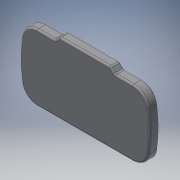
# Autodesk Inventor part: back cover
Saved by Autodesk Inventor 2019 (Build 230136000, 136)
## iProperties
Created: 2021-03-14
Part Number: back cover
Material: Generic
Document SubType Name: Modeling
Designer: Vijay
Density: 1 g/cm^3
Appearance: Default
Author: Vijay
Autodesk Inventor part; units mm, degrees
ref_plane "YZ Plane" through (0, 0, 0) normal (1, 0, 0) x (0, 1, 0)
ref_plane "XZ Plane" through (0, 0, 0) normal (0, 1, 0) x (-1, 0, 0)
ref_plane "XY Plane" through (0, 0, 0) normal (0, 0, 1) x (1, 0, 0)
sketch "Sketch1" plane through (0, 0, 0) normal (0, 0, 1) x (1, 0, 0)
  line L0 (-31.6571, 36.2117) -> (-28.1216, 39.7473) projected
  line L1 (-28.1216, 39.7473) -> (28.1216, 39.7473) projected
  line L2 (28.1216, 39.7473) -> (31.6571, 36.2117) projected
  arc A0 (31.6571, 36.2117) -> (35.1926, 34.7473) centre (35.1926, 39.7473) ccw projected
  line L3 (35.1926, 34.7473) -> (54.241, 34.7473) projected
  arc A1 (70.0672, 21.0991) -> (54.241, 34.7473) centre (54.241, 18.7473) ccw projected
  arc A2 (70.0672, -23.1161) -> (70.0672, 21.0991) centre (-78.6991, -1.0085) ccw projected
  arc A3 (54.241, -36.7642) -> (70.0672, -23.1161) centre (54.241, -20.7642) ccw projected
  line L4 (54.241, -36.7642) -> (-54.241, -36.7642) projected
  arc A4 (-70.0672, -23.1161) -> (-54.241, -36.7642) centre (-54.241, -20.7642) ccw projected
  arc A5 (-70.0672, 21.0991) -> (-70.0672, -23.1161) centre (78.6991, -1.0085) ccw projected
  arc A6 (-54.241, 34.7473) -> (-70.0672, 21.0991) centre (-54.241, 18.7473) ccw projected
  line L5 (-54.241, 34.7473) -> (-35.1926, 34.7473) projected
  arc A7 (-35.1926, 34.7473) -> (-31.6571, 36.2117) centre (-35.1926, 39.7473) ccw projected
  arc A8 (-27.7074, 41.7473) -> (-29.8287, 40.8686) centre (-27.7074, 38.7473) ccw projected
  line L6 (-29.8287, 40.8686) -> (-33.0713, 37.6259) projected
  arc A9 (-35.1926, 36.7473) -> (-33.0713, 37.6259) centre (-35.1926, 39.7473) ccw projected
  line L7 (-35.1926, 36.7473) -> (-54.241, 36.7473) projected
  arc A10 (-54.241, 36.7473) -> (-72.0455, 21.3931) centre (-54.241, 18.7473) ccw projected
  arc A11 (-72.0455, 21.3931) -> (-72.0455, -23.41) centre (78.6991, -1.0085) ccw projected
  arc A12 (-72.0455, -23.41) -> (-54.241, -38.7642) centre (-54.241, -20.7642) ccw projected
  line L8 (-54.241, -38.7642) -> (54.241, -38.7642) projected
  arc A13 (54.241, -38.7642) -> (72.0455, -23.41) centre (54.241, -20.7642) ccw projected
  arc A14 (72.0455, -23.41) -> (72.0455, 21.3931) centre (-78.6991, -1.0085) ccw projected
  arc A15 (72.0455, 21.3931) -> (54.241, 36.7473) centre (54.241, 18.7473) ccw projected
  line L9 (54.241, 36.7473) -> (35.1926, 36.7473) projected
  arc A16 (33.0713, 37.6259) -> (35.1926, 36.7473) centre (35.1926, 39.7473) ccw projected
  line L10 (33.0713, 37.6259) -> (29.8287, 40.8686) projected
  arc A17 (29.8287, 40.8686) -> (27.7074, 41.7473) centre (27.7074, 38.7473) ccw projected
  line L11 (27.7074, 41.7473) -> (-27.7074, 41.7473) projected
  line L12 (54.241, 32.7473) -> (35.1926, 32.7473) projected
  arc A18 (68.0889, 20.8051) -> (54.241, 32.7473) centre (54.241, 18.7473) ccw projected
  arc A19 (68.0889, -22.8221) -> (68.0889, 20.8051) centre (-78.6991, -1.0085) ccw projected
  arc A20 (54.241, -34.7642) -> (68.0889, -22.8221) centre (54.241, -20.7642) ccw projected
  line L13 (-54.241, -34.7642) -> (54.241, -34.7642) projected
  arc A21 (-68.0889, -22.8221) -> (-54.241, -34.7642) centre (-54.241, -20.7642) ccw projected
  arc A22 (-68.0889, 20.8051) -> (-68.0889, -22.8221) centre (78.6991, -1.0085) ccw projected
  arc A23 (-54.241, 32.7473) -> (-68.0889, 20.8051) centre (-54.241, 18.7473) ccw projected
  line L14 (-35.1926, 32.7473) -> (-54.241, 32.7473) projected
  arc A24 (-35.1926, 32.7473) -> (-30.2429, 34.7975) centre (-35.1926, 39.7473) ccw projected
  line L15 (-27.2931, 37.7473) -> (-30.2429, 34.7975) projected
  line L16 (27.2931, 37.7473) -> (-27.2931, 37.7473) projected
  line L17 (30.2429, 34.7975) -> (27.2931, 37.7473) projected
  arc A25 (30.2429, 34.7975) -> (35.1926, 32.7473) centre (35.1926, 39.7473) ccw projected
  line L18 (-28.1216, 39.7473) -> (28.1216, 39.7473) projected
  line L19 (-31.6571, 36.2117) -> (-28.1216, 39.7473) projected
  arc A26 (-35.1926, 34.7473) -> (-31.6571, 36.2117) centre (-35.1926, 39.7473) ccw projected
  line L20 (-54.241, 34.7473) -> (-35.1926, 34.7473) projected
  arc A27 (-54.241, 34.7473) -> (-70.0672, 21.0991) centre (-54.241, 18.7473) ccw projected
  arc A28 (-70.0672, 21.0991) -> (-70.0672, -23.1161) centre (78.6991, -1.0085) ccw projected
  arc A29 (-70.0672, -23.1161) -> (-54.241, -36.7642) centre (-54.241, -20.7642) ccw projected
  line L21 (54.241, -36.7642) -> (-54.241, -36.7642) projected
  arc A30 (54.241, -36.7642) -> (70.0672, -23.1161) centre (54.241, -20.7642) ccw projected
  arc A31 (70.0672, -23.1161) -> (70.0672, 21.0991) centre (-78.6991, -1.0085) ccw projected
  arc A32 (70.0672, 21.0991) -> (54.241, 34.7473) centre (54.241, 18.7473) ccw projected
  line L22 (35.1926, 34.7473) -> (54.241, 34.7473) projected
  arc A33 (31.6571, 36.2117) -> (35.1926, 34.7473) centre (35.1926, 39.7473) ccw projected
  line L23 (28.1216, 39.7473) -> (31.6571, 36.2117) projected
  point P0 (0, 0)
extrude "Extrusion1" add sketch "Sketch1" along normal blind 8 contours L0 L1 L2 A0 L3 A1 A2 A3 L4 A4 A5 A6 L5 A7 | L11 A17 L10 A16 L9 A15 A14 A13 L8 A12 A11 A10 L7 A9 L6 A8
sketch "Sketch2" plane through (0, 0, 8) normal (0, 0, 1) x (1, 0, 0)
  arc A0 (68.0889, 20.8051) -> (54.241, 32.7473) centre (54.241, 18.7473) ccw projected
  arc A1 (68.0889, -22.8221) -> (68.0889, 20.8051) centre (-78.6991, -1.0085) ccw projected
  arc A2 (54.241, -34.7642) -> (68.0889, -22.8221) centre (54.241, -20.7642) ccw projected
  line L0 (54.241, -34.7642) -> (-54.241, -34.7642) projected
  arc A3 (-68.0889, -22.8221) -> (-54.241, -34.7642) centre (-54.241, -20.7642) ccw projected
  arc A4 (-68.0889, 20.8051) -> (-68.0889, -22.8221) centre (78.6991, -1.0085) ccw projected
  arc A5 (-54.241, 32.7473) -> (-68.0889, 20.8051) centre (-54.241, 18.7473) ccw projected
  line L1 (-54.241, 32.7473) -> (-35.1926, 32.7473) projected
  arc A6 (-35.1926, 32.7473) -> (-30.2429, 34.7975) centre (-35.1926, 39.7473) ccw projected
  line L2 (-30.2429, 34.7975) -> (-27.2931, 37.7473) projected
  line L3 (-27.2931, 37.7473) -> (27.2931, 37.7473) projected
  line L4 (27.2931, 37.7473) -> (30.2429, 34.7975) projected
  arc A7 (30.2429, 34.7975) -> (35.1926, 32.7473) centre (35.1926, 39.7473) ccw projected
  line L5 (35.1926, 32.7473) -> (54.241, 32.7473) projected
  arc A8 (-27.7074, 41.7473) -> (-29.8287, 40.8686) centre (-27.7074, 38.7473) ccw projected
  line L6 (-29.8287, 40.8686) -> (-33.0713, 37.6259) projected
  arc A9 (-35.1926, 36.7473) -> (-33.0713, 37.6259) centre (-35.1926, 39.7473) ccw projected
  line L7 (-35.1926, 36.7473) -> (-54.241, 36.7473) projected
  arc A10 (-54.241, 36.7473) -> (-72.0455, 21.3931) centre (-54.241, 18.7473) ccw projected
  arc A11 (-72.0455, 21.3931) -> (-72.0455, -23.41) centre (78.6991, -1.0085) ccw projected
  arc A12 (-72.0455, -23.41) -> (-54.241, -38.7642) centre (-54.241, -20.7642) ccw projected
  line L8 (-54.241, -38.7642) -> (54.241, -38.7642) projected
  arc A13 (54.241, -38.7642) -> (72.0455, -23.41) centre (54.241, -20.7642) ccw projected
  arc A14 (72.0455, -23.41) -> (72.0455, 21.3931) centre (-78.6991, -1.0085) ccw projected
  arc A15 (72.0455, 21.3931) -> (54.241, 36.7473) centre (54.241, 18.7473) ccw projected
  line L9 (54.241, 36.7473) -> (35.1926, 36.7473) projected
  arc A16 (33.0713, 37.6259) -> (35.1926, 36.7473) centre (35.1926, 39.7473) ccw projected
  line L10 (33.0713, 37.6259) -> (29.8287, 40.8686) projected
  arc A17 (29.8287, 40.8686) -> (27.7074, 41.7473) centre (27.7074, 38.7473) ccw projected
  line L11 (27.7074, 41.7473) -> (-27.7074, 41.7473) projected
  point P0 (0, 0)
extrude "Extrusion2" add sketch "Sketch2" along normal blind 2 contours A1 A2 L0 A3 A4 A5 L1 A6 L2 L3 L4 A7 L5 A0 | L11 A17 L10 A16 L9 A15 A14 A13 L8 A12 A11 A10 L7 A9 L6 A8
fillet "Fillet1" radius 2 29 edges at (-65.9963, -34.3955, 10) (0, -38.7642, 10) (65.9963, -34.3955, 10) (73.7009, -1.0085, 10) (65.9963, 32.3786, 10) (44.7168, 36.7473, 10) (34.0446, 36.9756, 10) (31.45, 39.2473, 10) (28.8554, 41.5189, 10) (0, 41.7473, 10) (-28.8554, 41.5189, 10) (-31.45, 39.2473, 10) (-34.0446, 36.9756, 10) (-44.7168, 36.7473, 10) (-65.9963, 32.3786, 10) (-73.7009, -1.0085, 10) (-44.7168, 32.7473, 8) (-32.5139, 33.2801, 8) (-28.768, 36.2724, 8) (-69.7009, -1.0085, 8) (-63.384, -31.3663, 8) (0, -34.7642, 8) (63.384, -31.3663, 8) (69.7009, -1.0085, 8) (63.384, 29.3494, 8) (44.7168, 32.7473, 8) (32.5139, 33.2801, 8) (28.768, 36.2724, 8) (-63.384, 29.3494, 8)
sketch "Sketch3" plane through (0, 0, 0) normal (0, 0, -1) x (-1, 0, 0)
  line L0 (31.6571, 36.2117) -> (28.1216, 39.7473) projected
  line L1 (28.1216, 39.7473) -> (-28.1216, 39.7473) projected
  line L2 (-28.1216, 39.7473) -> (-31.6571, 36.2117) projected
  arc A0 (-35.1926, 34.7473) -> (-31.6571, 36.2117) centre (-35.1926, 39.7473) ccw projected
  line L3 (-35.1926, 34.7473) -> (-54.241, 34.7473) projected
  arc A1 (-54.241, 34.7473) -> (-70.0672, 21.0991) centre (-54.241, 18.7473) ccw projected
  arc A2 (-70.0672, 21.0991) -> (-70.0672, -23.1161) centre (78.6991, -1.0085) ccw projected
  arc A3 (-70.0672, -23.1161) -> (-54.241, -36.7642) centre (-54.241, -20.7642) ccw projected
  line L4 (-54.241, -36.7642) -> (54.241, -36.7642) projected
  arc A4 (54.241, -36.7642) -> (70.0672, -23.1161) centre (54.241, -20.7642) ccw projected
  arc A5 (70.0672, -23.1161) -> (70.0672, 21.0991) centre (-78.6991, -1.0085) ccw projected
  arc A6 (70.0672, 21.0991) -> (54.241, 34.7473) centre (54.241, 18.7473) ccw projected
  line L5 (54.241, 34.7473) -> (35.1926, 34.7473) projected
  arc A7 (31.6571, 36.2117) -> (35.1926, 34.7473) centre (35.1926, 39.7473) ccw projected
  arc A8 (29.8287, 40.8686) -> (27.7074, 41.7473) centre (27.7074, 38.7473) ccw projected
  line L6 (29.8287, 40.8686) -> (33.0713, 37.6259) projected
  arc A9 (33.0713, 37.6259) -> (35.1926, 36.7473) centre (35.1926, 39.7473) ccw projected
  line L7 (35.1926, 36.7473) -> (54.241, 36.7473) projected
  arc A10 (72.0455, 21.3931) -> (54.241, 36.7473) centre (54.241, 18.7473) ccw projected
  arc A11 (72.0455, -23.41) -> (72.0455, 21.3931) centre (-78.6991, -1.0085) ccw projected
  arc A12 (54.241, -38.7642) -> (72.0455, -23.41) centre (54.241, -20.7642) ccw projected
  line L8 (54.241, -38.7642) -> (-54.241, -38.7642) projected
  arc A13 (-72.0455, -23.41) -> (-54.241, -38.7642) centre (-54.241, -20.7642) ccw projected
  arc A14 (-72.0455, 21.3931) -> (-72.0455, -23.41) centre (78.6991, -1.0085) ccw projected
  arc A15 (-54.241, 36.7473) -> (-72.0455, 21.3931) centre (-54.241, 18.7473) ccw projected
  line L9 (-54.241, 36.7473) -> (-35.1926, 36.7473) projected
  arc A16 (-35.1926, 36.7473) -> (-33.0713, 37.6259) centre (-35.1926, 39.7473) ccw projected
  line L10 (-33.0713, 37.6259) -> (-29.8287, 40.8686) projected
  arc A17 (-27.7074, 41.7473) -> (-29.8287, 40.8686) centre (-27.7074, 38.7473) ccw projected
  line L11 (-27.7074, 41.7473) -> (27.7074, 41.7473) projected
  arc A18 (-54.241, 32.7473) -> (-68.0889, 20.8051) centre (-54.241, 18.7473) ccw projected
  line L12 (-54.241, 32.7473) -> (-35.1926, 32.7473) projected
  arc A19 (-35.1926, 32.7473) -> (-30.2429, 34.7975) centre (-35.1926, 39.7473) ccw projected
  line L13 (-30.2429, 34.7975) -> (-27.2931, 37.7473) projected
  line L14 (-27.2931, 37.7473) -> (27.2931, 37.7473) projected
  line L15 (27.2931, 37.7473) -> (30.2429, 34.7975) projected
  arc A20 (30.2429, 34.7975) -> (35.1926, 32.7473) centre (35.1926, 39.7473) ccw projected
  line L16 (35.1926, 32.7473) -> (54.241, 32.7473) projected
  arc A21 (68.0889, 20.8051) -> (54.241, 32.7473) centre (54.241, 18.7473) ccw projected
  arc A22 (68.0889, -22.8221) -> (68.0889, 20.8051) centre (-78.6991, -1.0085) ccw projected
  arc A23 (54.241, -34.7642) -> (68.0889, -22.8221) centre (54.241, -20.7642) ccw projected
  line L17 (54.241, -34.7642) -> (-54.241, -34.7642) projected
  arc A24 (-68.0889, -22.8221) -> (-54.241, -34.7642) centre (-54.241, -20.7642) ccw projected
  arc A25 (-68.0889, 20.8051) -> (-68.0889, -22.8221) centre (78.6991, -1.0085) ccw projected
  arc A26 (29.8287, 40.8686) -> (27.7074, 41.7473) centre (27.7074, 38.7473) ccw projected
  line L18 (-27.7074, 41.7473) -> (27.7074, 41.7473) projected
  arc A27 (-27.7074, 41.7473) -> (-29.8287, 40.8686) centre (-27.7074, 38.7473) ccw projected
  line L19 (-33.0713, 37.6259) -> (-29.8287, 40.8686) projected
  arc A28 (-35.1926, 36.7473) -> (-33.0713, 37.6259) centre (-35.1926, 39.7473) ccw projected
  line L20 (-54.241, 36.7473) -> (-35.1926, 36.7473) projected
  arc A29 (-54.241, 36.7473) -> (-72.0455, 21.3931) centre (-54.241, 18.7473) ccw projected
  arc A30 (-72.0455, 21.3931) -> (-72.0455, -23.41) centre (78.6991, -1.0085) ccw projected
  arc A31 (-72.0455, -23.41) -> (-54.241, -38.7642) centre (-54.241, -20.7642) ccw projected
  line L21 (54.241, -38.7642) -> (-54.241, -38.7642) projected
  arc A32 (54.241, -38.7642) -> (72.0455, -23.41) centre (54.241, -20.7642) ccw projected
  arc A33 (72.0455, -23.41) -> (72.0455, 21.3931) centre (-78.6991, -1.0085) ccw projected
  arc A34 (72.0455, 21.3931) -> (54.241, 36.7473) centre (54.241, 18.7473) ccw projected
  line L22 (35.1926, 36.7473) -> (54.241, 36.7473) projected
  arc A35 (33.0713, 37.6259) -> (35.1926, 36.7473) centre (35.1926, 39.7473) ccw projected
  line L23 (29.8287, 40.8686) -> (33.0713, 37.6259) projected
  point P0 (0, 0)
extrude "Extrusion3" add sketch "Sketch3" along normal blind 1.8 contours A7 L5 A6 A5 A4 L4 A3 A2 A1 L3 A0 L2 L1 L0
sketch "Sketch4" plane through (0, 0, -1.8) normal (0, 0, -1) x (-1, 0, 0)
  line L0 (-54.241, 32.7473) -> (-35.1926, 32.7473) projected
  arc A0 (-54.241, 32.7473) -> (-68.0889, 20.8051) centre (-54.241, 18.7473) ccw projected
  arc A1 (-68.0889, 20.8051) -> (-68.0889, -22.8221) centre (78.6991, -1.0085) ccw projected
  arc A2 (-68.0889, -22.8221) -> (-54.241, -34.7642) centre (-54.241, -20.7642) ccw projected
  line L1 (54.241, -34.7642) -> (-54.241, -34.7642) projected
  arc A3 (54.241, -34.7642) -> (68.0889, -22.8221) centre (54.241, -20.7642) ccw projected
  arc A4 (68.0889, -22.8221) -> (68.0889, 20.8051) centre (-78.6991, -1.0085) ccw projected
  arc A5 (68.0889, 20.8051) -> (54.241, 32.7473) centre (54.241, 18.7473) ccw projected
  line L2 (35.1926, 32.7473) -> (54.241, 32.7473) projected
  arc A6 (30.2429, 34.7975) -> (35.1926, 32.7473) centre (35.1926, 39.7473) ccw projected
  line L3 (27.2931, 37.7473) -> (30.2429, 34.7975) projected
  line L4 (-27.2931, 37.7473) -> (27.2931, 37.7473) projected
  line L5 (-30.2429, 34.7975) -> (-27.2931, 37.7473) projected
  arc A7 (-35.1926, 32.7473) -> (-30.2429, 34.7975) centre (-35.1926, 39.7473) ccw projected
  line L6 (28.1216, 39.7473) -> (-28.1216, 39.7473) projected
  line L7 (31.6571, 36.2117) -> (28.1216, 39.7473) projected
  arc A8 (31.6571, 36.2117) -> (35.1926, 34.7473) centre (35.1926, 39.7473) ccw projected
  line L8 (54.241, 34.7473) -> (35.1926, 34.7473) projected
  arc A9 (70.0672, 21.0991) -> (54.241, 34.7473) centre (54.241, 18.7473) ccw projected
  arc A10 (70.0672, -23.1161) -> (70.0672, 21.0991) centre (-78.6991, -1.0085) ccw projected
  arc A11 (54.241, -36.7642) -> (70.0672, -23.1161) centre (54.241, -20.7642) ccw projected
  line L9 (-54.241, -36.7642) -> (54.241, -36.7642) projected
  arc A12 (-70.0672, -23.1161) -> (-54.241, -36.7642) centre (-54.241, -20.7642) ccw projected
  arc A13 (-70.0672, 21.0991) -> (-70.0672, -23.1161) centre (78.6991, -1.0085) ccw projected
  arc A14 (-54.241, 34.7473) -> (-70.0672, 21.0991) centre (-54.241, 18.7473) ccw projected
  line L10 (-35.1926, 34.7473) -> (-54.241, 34.7473) projected
  arc A15 (-35.1926, 34.7473) -> (-31.6571, 36.2117) centre (-35.1926, 39.7473) ccw projected
  line L11 (-28.1216, 39.7473) -> (-31.6571, 36.2117) projected
  arc A16 (69.6715, -23.0573) -> (69.6715, 21.0403) centre (-78.6991, -1.0085) ccw
  arc A17 (69.6715, 21.0403) -> (54.241, 34.3473) centre (54.241, 18.7473) ccw
  line L12 (54.241, 34.3473) -> (35.1926, 34.3473)
  arc A18 (31.3743, 35.9289) -> (35.1926, 34.3473) centre (35.1926, 39.7473) ccw
  line L13 (31.3743, 35.9289) -> (27.9559, 39.3473)
  line L14 (27.9559, 39.3473) -> (-27.9559, 39.3473)
  line L15 (-27.9559, 39.3473) -> (-31.3743, 35.9289)
  arc A19 (-35.1926, 34.3473) -> (-31.3743, 35.9289) centre (-35.1926, 39.7473) ccw
  line L16 (-35.1926, 34.3473) -> (-54.241, 34.3473)
  arc A20 (-54.241, 34.3473) -> (-69.6715, 21.0403) centre (-54.241, 18.7473) ccw
  arc A21 (-69.6715, 21.0403) -> (-69.6715, -23.0573) centre (78.6991, -1.0085) ccw
  arc A22 (-69.6715, -23.0573) -> (-54.241, -36.3642) centre (-54.241, -20.7642) ccw
  line L17 (-54.241, -36.3642) -> (54.241, -36.3642)
  arc A23 (54.241, -36.3642) -> (69.6715, -23.0573) centre (54.241, -20.7642) ccw
  point P0 (0, 0)
  dimension "d7" = 0.4
  constraints: 16 point on circle, 12 end point, 8 centre point, 13 other
  measures "d7" radial gap between concentric circles of A11 A23
extrude "Extrusion4" cut sketch "Sketch4" against normal blind 1.8 contours L7 A8 L8 A9 A10 A11 L9 A12 A13 A14 L10 A15 L11 L6
chamfer "Chamfer1" distance 0.5 angle 45 14 edges at (0, -36.3642, -1.8) (-64.4289, -32.578, -1.8) (-71.3009, -1.0085, -1.8) (-64.4289, 30.5611, -1.8) (-44.7168, 34.3473, -1.8) (-33.1262, 34.7583, -1.8) (-29.6651, 37.6381, -1.8) (64.4289, -32.578, -1.8) (71.3009, -1.0085, -1.8) (64.4289, 30.5611, -1.8) (44.7168, 34.3473, -1.8) (33.1262, 34.7583, -1.8) (29.6651, 37.6381, -1.8) (0, 39.3473, -1.8)
chamfer "Chamfer2" distance 0.5 angle 45 16 edges at (-65.9963, 32.3786, 0) (-73.7009, -1.0085, 0) (-65.9963, -34.3955, 0) (0, -38.7642, 0) (65.9963, -34.3955, 0) (73.7009, -1.0085, 0) (65.9963, 32.3786, 0) (44.7168, 36.7473, 0) (34.0446, 36.9756, 0) (31.45, 39.2473, 0) (28.8554, 41.5189, 0) (0, 41.7473, 0) (-28.8554, 41.5189, 0) (-31.45, 39.2473, 0) (-34.0446, 36.9756, 0) (-44.7168, 36.7473, 0)
sketch "Sketch5" plane through (-54.241, -38.7642, 8) normal (0, -1, 0) x (1, 0, 0)
  line L0 (96.8896, -5.35) -> (96.8894, -5.35) projected
  line L1 (96.8837, -5.35) -> (96.8894, -5.35) projected
  line L2 (96.8837, -5.35) -> (96.8837, -2.35) projected
  line L3 (96.8896, -2.35) -> (96.8837, -2.35) projected
  line L4 (96.8896, -5.35) -> (96.8896, -2.35) projected
  line L5 (87.4787, -5.35) -> (87.4787, -2.35) projected
  line L6 (98.5846, -1.2991) -> (86.2743, -1.2991)
  line L7 (86.2743, -1.2991) -> (86.2743, -10.4423)
  line L8 (86.2743, -10.4423) -> (98.5846, -10.4423)
  line L9 (98.5846, -10.4423) -> (98.5846, -1.2991)
  point P0 (54.241, -8)
  constraints: 8 end point, 2 parallel, 1 horizontal, 1 perpendicular
extrude "Extrusion5" cut sketch "Sketch5" against normal blind 17.45 contours L2 L3 L4 L1 | L9 L8 L7 L6
fillet "Fillet2" radius 2 2 edges at (44.3437, -36.7008, 6.7009) (32.0334, -36.7008, 6.7009)
chamfer "Chamfer4" distance 2 angle 45 5 edges at (43.7579, -38.7642, 6.1151) (38.1885, -38.7642, 6.7009) (32.6192, -38.7642, 6.1151) (32.0334, -38.7642, 2.6004) (44.3437, -38.7642, 2.6004)
body "Solid1"
